Autodesk Inventor part; units mm, degrees
(part 18 of 18)
sketch "Sketch18" plane through (0, 13.762, -7.5) normal (0, 1, 0) x (1, 0, 0)
  line L0 (-9.984, -8.484) -> (-9.984, 31.4609) projected
  line L1 (-9.984, 31.4609) -> (9.984, 31.4609) projected
  line L2 (9.984, 31.4609) -> (9.984, -8.484) projected
  line L3 (9.984, -8.484) -> (-9.984, -8.484) projected
  line L4 (11, -9.5) -> (11, 32.4769) projected
  line L5 (11, 32.4769) -> (-11, 32.4769) projected
  line L6 (-11, 32.4769) -> (-11, -9.5) projected
  line L7 (-11, -9.5) -> (11, -9.5) projected
  point P0 (0, -7.5)
  point P1 (-9.984, -7.5)
  point P2 (9.984, -7.5)
extrude "Extrusion13" add sketch "Sketch18" along normal blind 12 draft 6
sketch "Sketch19" plane through (0, 25.762, -7.5) normal (0, 1, 0) x (1, 0, 0)
  line L0 (-10.7373, 31.7382) -> (10.527, 31.7382)
  line L1 (10.527, 31.7382) -> (10.527, -9.2373)
  line L2 (10.527, -9.2373) -> (-10.7373, -9.2373)
  line L3 (-10.7373, -9.2373) -> (-10.7373, 31.7382)
  line L4 (-12.2613, 33.7382) -> (12.2613, 33.7382) projected
  line L5 (12.2613, -10.7613) -> (-12.2613, -10.7613) projected
  line L6 (-12.2613, -10.7613) -> (-12.2613, 33.7382) projected
  point P0 (0, -7.5)
  point P1 (-0.1051, 31.7382)
  point P2 (-0.1051, 30.8661)
  dimension "d183" = 2
  dimension "d184" = 1.524
  dimension "d185" = 1.524
  constraints: 8 end point, 2 parallel, 1 horizontal, 1 midpoint, 1 perpendicular, 1 vertical alignment
  measures "d183" distance between parallel lines of L0 L4
  measures "d184" distance between parallel lines of L5 L2
  measures "d185" distance between parallel lines of L3 L6
sketch "Sketch20" plane through (0, 13.762, -7.5) normal (0, 1, 0) x (-1, 0, 0)
  line L0 (9.984, 8.484) -> (-9.984, 8.484)
  line L1 (-9.984, 8.484) -> (-9.984, -31.4609)
  line L2 (-9.984, -31.4609) -> (9.984, -31.4609)
  line L3 (9.984, -31.4609) -> (9.984, 8.484)
  point P0 (0, 7.5)
  constraints: 8 end point, 2 parallel, 1 coincident, 1 horizontal, 1 perpendicular
loft "Loft1" cut profiles "Sketch20", "Sketch19"
ref_plane "Work Plane11" through (0, 0, -53) normal (0, 0, -1) x (-1, 0, 0)
sketch "Sketch45" plane through (0, 25.762, -41.2382) normal (0, 0.9876883, 0.1564345) x (1, 0, 0)
  line L0 (-21.726, 2.2802) -> (18.9133, 2.2802)
  line L1 (18.9133, 2.2802) -> (18.9133, -50.289)
  line L2 (18.9133, -50.289) -> (-21.726, -50.289)
  line L3 (-21.726, -50.289) -> (-21.726, 2.2802)
  point P0 (0, 0)
  constraints: 8 end point, 2 parallel, 1 horizontal, 1 perpendicular
extrude "Extrusion22" cut sketch "Sketch45" along normal through all
sketch "Sketch46" plane through (0, 25.762, -41.2382) normal (0, 0.9876883, 0.1564345) x (1, 0, 0)
  line L0 (0, 130.5778) -> (0, -158.8957) projected
  line L1 (-11.5326, -44.3164) -> (-12.2613, 0) projected
  line L2 (12.2613, 0) -> (11.5326, -44.3164) projected
  line L3 (11.5326, -44.3164) -> (-11.5326, -44.3164) projected
  line L4 (-12.2613, 0) -> (12.2613, 0) projected
  line L5 (-10.783, -1) -> (10.783, -1)
  line L6 (10.783, -1) -> (10.783, -43.5544)
  line L7 (10.783, -43.5544) -> (-10.783, -43.5544)
  line L8 (-10.783, -43.5544) -> (-10.783, -1)
  point P0 (0, -1)
  point P1 (0, 0)
  dimension "d265" = 1
  dimension "d266" = 0.762
  dimension "d267" = 0.762
  constraints: 8 end point, 2 midpoint, 2 parallel, 1 horizontal, 1 perpendicular, 1 vertical alignment
  measures "d265" distance between parallel lines of L4 L5
  measures "d266" distance from line of L3 L6.end
  measures "d267" distance from line of L1 L7.end
extrude "Extrusion23" cut sketch "Sketch46" against normal blind 0.762 contours L5 L6 L7 L0 | L0 L7 L8 L5
sketch "Sketch47" plane through (0, 13.762, -7.5) normal (0, 1, 0) x (-1, 0, 0)
  spline S0 degree 4 poles (-11, 9.5) (-11, 10.8469) (-10.4161, 12.7101) (-9.67, 17.8605) (-2.21, 18.1401) (-1.3548, 20.0653) (0, 20.0653) knots 0 0 0 0 0 0.372809 0.622809 1 1 1 1 1
  line L0 (11, 9.5) -> (-11, 9.5)
  spline S1 degree 4 poles (11, 9.5) (11, 10.8469) (10.4161, 12.7101) (9.6698, 17.8603) (2.21, 18.1401) (1.3548, 20.0653) (0, 20.0653) knots 0 0 0 0 0 0.37281 0.62281 1 1 1 1 1
  line L1 (0, 20.0653) -> (3.3697, 20.0653)
  line L2 (-11, 9.5) -> (11, 9.5) projected
  line L3 (-11, 7.5) -> (-11, 9.5) projected
  line L4 (11, 9.5) -> (11, 7.5) projected
  line L5 (0, 20.0653) -> (-2.678, 20.0653)
  point P0 (0, 7.5)
  point P1 (-10.4676, 12.6318)
  point P2 (-8.1795, 16.4094)
  point P3 (-2.678, 18.88)
  point P4 (10.4676, 12.6318)
  point P5 (8.1793, 16.4093)
  point P6 (2.678, 18.88)
  point P7 (-10.2, 9.5)
  point P8 (10.1999, 9.5)
  point P9 (0, 9.5)
  constraints: 6 end point, 2 horizontal, 2 point on line, 2 vertical, 1 midpoint, 1 parallel, 1 perpendicular, 10 other
extrude "Extrusion24" add sketch "Sketch47" against normal up to next
sketch "Sketch48" plane through (0, 25.762, -41.2382) normal (0, 0.9876883, 0.1564345) x (1, 0, 0)
  spline S0 degree 4 poles (-11.5326, -44.3164) (-11.5144, -45.4246) (-8.7357, -45.2988) (-4.4271, -45.9469) (-1.7264, -46.8919) (0, -46.8919) knots 0 0 0 0 0 0.464328 1 1 1 1 1
  spline S1 degree 4 poles (11.5326, -44.3164) (11.5144, -45.4246) (8.7357, -45.2988) (4.4271, -45.9469) (1.7264, -46.8919) (0, -46.8919) knots 0 0 0 0 0 0.464328 1 1 1 1 1
  line L0 (-11.5326, -44.3164) -> (11.5326, -44.3164)
  point P0 (0, -44.7605)
  point P1 (-10.0361, -45.361)
  point P2 (-4.7135, -46.095)
  point P3 (10.0361, -45.361)
  point P4 (4.7135, -46.095)
  constraints: 2 end point, 8 other
sketch "Sketch49" plane through (0, 13.762, -7.5) normal (0, 1, 0) x (1, 0, 0)
  arc A0 (-11, -9.5) -> (0, -20.0653) centre (0, -20.0653) ccw projected
  arc A1 (0, -20.0653) -> (11, -9.5) centre (11, -9.5) ccw projected
  line L0 (-11, -9.5) -> (11, -9.5) projected
  point P0 (0, -7.5)
  constraints: 2 other
loft "Loft8" add profiles "Sketch48" section 1 edges at (-7.9061, 13.762, 9.1062) (7.9063, 13.762, 9.1063) (0, 13.762, 2)
sketch "Sketch50" plane through (0, 13.762, -7.5) normal (0, 1, 0) x (-1, 0, 0)
  spline S0 degree 4 poles (0, 20.0653) (-1.3548, 20.0653) (-2.21, 18.1401) (-9.67, 17.8605) (-10.4161, 12.7101) (-11, 10.8469) (-11, 9.5) knots 0 0 0 0 0 0.377191 0.627191 1 1 1 1 1 projected
  spline S1 degree 4 poles (11, 9.5) (11, 10.8469) (10.4161, 12.7101) (9.6698, 17.8603) (2.21, 18.1401) (1.3548, 20.0653) (0, 20.0653) knots 0 0 0 0 0 0.37281 0.62281 1 1 1 1 1 projected
  line L0 (9.984, 8.484) -> (-9.984, 8.484) projected
  line L1 (9.984, 10.4474) -> (9.984, 8.484)
  line L2 (-9.984, 8.484) -> (-9.984, 10.4474)
  line L3 (-11, 7.5) -> (-11, 9.5) projected
  line L4 (-9.8386, 8.484) -> (9.984, 8.484)
  spline S2 degree 5 poles (-9.984, 10.4474) (-9.9761, 10.5053) (-9.9677, 10.5633) (-9.9589, 10.6211) (-9.9066, 10.9478) (-9.8414, 11.2723) (-9.7813, 11.538) (-9.6438, 12.0907) (-9.4804, 12.6364) (-9.3877, 12.9187) (-9.1847, 13.4787) (-8.9361, 14.0199) (-8.7984, 14.285) (-8.4835, 14.7998) (-8.0862, 15.2544) (-7.8638, 15.4637) (-7.3377, 15.8789) (-6.7522, 16.2068) (-6.4221, 16.3641) (-5.7049, 16.6687) (-4.9708, 16.9302) (-4.5802, 17.0664) (-3.8287, 17.3363) (-3.0886, 17.6355) (-2.7363, 17.7905) (-2.1263, 18.0862) (-1.5364, 18.4207) (-1.284, 18.5692) (-0.8949, 18.8138) (-0.4841, 19.0178) (-0.3319, 19.0855) (-0.1652, 19.1191) (0, 19.118) knots 0 0 0 0 0 0 0.020521 0.020521 0.020521 0.116026 0.116026 0.116026 0.220222 0.220222 0.220222 0.324743 0.324743 0.324743 0.431166 0.431166 0.431166 0.559208 0.559208 0.559208 0.704346 0.704346 0.704346 0.839163 0.839163 0.839163 0.942014 0.942014 0.942014 1 1 1 1 1 1
  spline S3 degree 5 poles (0, 19.118) (0.1652, 19.1191) (0.3319, 19.0855) (0.4841, 19.0178) (0.8948, 18.8138) (1.2839, 18.5693) (1.5363, 18.4207) (2.1262, 18.0862) (2.7363, 17.7905) (3.0885, 17.6355) (3.8286, 17.3362) (4.5801, 17.0663) (4.9707, 16.9301) (5.7048, 16.6687) (6.422, 16.3641) (6.752, 16.2067) (7.3375, 15.8788) (7.8637, 15.4636) (8.086, 15.2543) (8.4834, 14.7997) (8.7983, 14.2849) (8.936, 14.0198) (9.1846, 13.4786) (9.3877, 12.9186) (9.4804, 12.6363) (9.6437, 12.0906) (9.7813, 11.5379) (9.8413, 11.2722) (9.9065, 10.9477) (9.9589, 10.6211) (9.9677, 10.5632) (9.9761, 10.5053) (9.984, 10.4474) knots 0 0 0 0 0 0 0.057985 0.057985 0.057985 0.160835 0.160835 0.160835 0.295652 0.295652 0.295652 0.440789 0.440789 0.440789 0.568833 0.568833 0.568833 0.675258 0.675258 0.675258 0.77978 0.77978 0.77978 0.883976 0.883976 0.883976 0.97948 0.97948 0.97948 1 1 1 1 1 1
  point P0 (0, 7.5)
  constraints: 6 end point, 1 parallel, 1 perpendicular, 1 point on line, 6 other
extrude "Extrusion26" cut sketch "Sketch50" against normal up to next
equation "\"d22\" = d24"
equation "\"d23\" = d24"
equation "\"d37\" = t"
equation "\"d40\" = t"
equation "\"t\" = 1.016"
equation "\"d14\" = d24"
equation "\"d24\" = 1.016"
body "Solid1"
